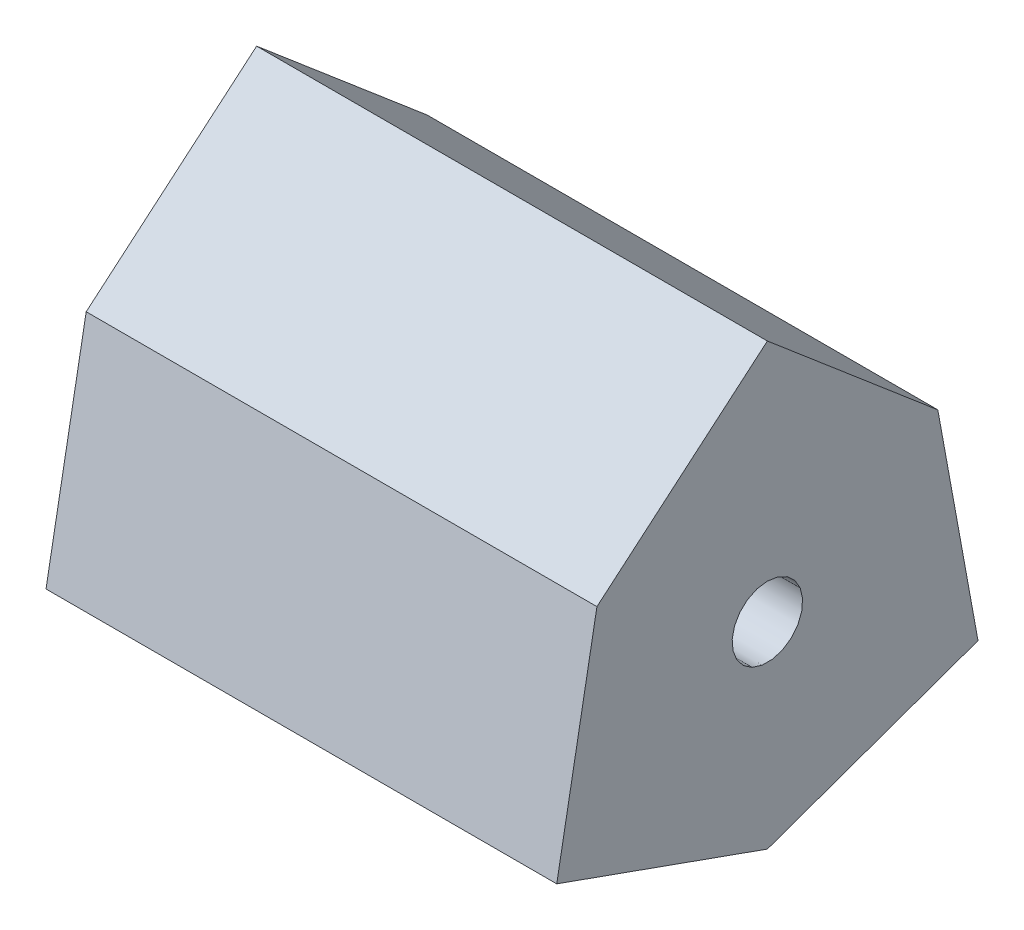
# Autodesk Inventor part: eje motor
Saved by Autodesk Inventor 2016 (Build 200138000, 138)
## iProperties
Created: 2016-06-25
Part Number: eje motor
Material: Generic
Document SubType Name: Modeling
Designer: Admin
Density: 1 g/cm^3
Appearance: Default
Author: Admin
Autodesk Inventor part; units mm, degrees
ref_plane "YZ Plane" through (0, 0, 0) normal (1, 0, 0) x (0, 1, 0)
ref_plane "XZ Plane" through (0, 0, 0) normal (0, 1, 0) x (-1, 0, 0)
ref_plane "XY Plane" through (0, 0, 0) normal (0, 0, 1) x (1, 0, 0)
sketch "Block1" plane through (0, 0, 0) normal (0, 0, 1) x (1, 0, 0)
  line L0 (4.046, 7.0078) -> (10, 0)
  line L1 (4.046, -7.0078) -> (10, 0)
  line L2 (4.046, -7.0078) -> (-5, -8.6603)
  line L3 (-5, -8.6603) -> (-8.092, 0)
  line L4 (-8.092, 0) -> (-5, 8.6603)
  line L5 (-5, 8.6603) -> (4.046, 7.0078)
  point P0 (0, 0)
sketch "Sketch1" plane through (0, 0, 0) normal (1, 0, 0) x (0, 1, 0)
  circle A0 centre (0, 0) radius 1.45
  line L0 (4.046, 7.0078) -> (10, 0)
  line L1 (4.046, -7.0078) -> (10, 0)
  line L2 (4.046, -7.0078) -> (-5, -8.6603)
  line L3 (-5, -8.6603) -> (-8.092, 0)
  line L4 (-8.092, 0) -> (-5, 8.6603)
  line L5 (-5, 8.6603) -> (4.046, 7.0078)
  point P0 (-0.5025, 0)
  point P1 (-0.5025, 0)
  dimension "d3" = 2.9
  constraints: 9 coincident, 1 centre point
  measures "d3" diameter of A0
extrude "Extrusion1" add sketch "Sketch1" along normal blind 21
body "Solid1"
